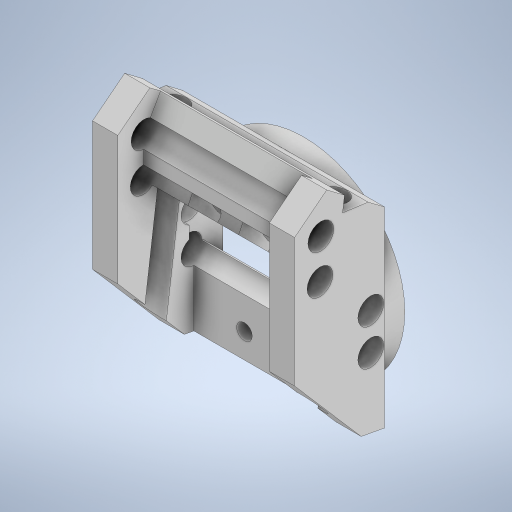
# Autodesk Inventor part: arm_head_top
Saved by Autodesk Inventor 2023.4 (Build 274418000, 418)
## iProperties
Created: 2024-03-10
Part Number: arm_head_top
Material: Generic
Document SubType Name: Modeling
Designer: aaron
Density: 1 g/cm^3
Appearance: Default
Author: aaron
Autodesk Inventor part; units mm, degrees
ref_plane "YZ Plane" through (0, 0, 0) normal (1, 0, 0) x (0, 1, 0)
ref_plane "XZ Plane" through (0, 0, 0) normal (0, 1, 0) x (-1, 0, 0)
sketch "Sketch1" plane through (0, 0, 0) normal (0, 0, 1) x (1, 0, 0)
  circle A0 centre (0, 0) radius 20
  dimension "d0" = 40
  constraints: 1 centre point, 1 coincident
  measures "d0" diameter of A0
extrude "Extrusion1" add sketch "Sketch1" along normal blind 4
sketch "Sketch2" plane through (0, 0, 0) normal (1, 0, 0) x (0, 1, 0)
  circle A0 centre (3.6, 6.738761) radius 2.55
  circle A1 centre (13.561537, 16.796235) radius 2.55
  circle A2 centre (21.281943, 16.626298) radius 2.55
  line L0 (20, 4) -> (-20, 4)
  line L1 (20, 4) -> (28.645843, 15.452424)
  line L2 (28.645843, 15.452424) -> (23.66832, 21.807503)
  circle A3 centre (-3.6, 6.738761) radius 2.55
  line L3 (23.66832, 21.807503) -> (-1.788198, 21.807503)
  line L4 (-1.788198, 21.807503) -> (-17.016826, 8.639245)
  line L5 (-17.016826, 8.639245) -> (-17.886444, 4)
  line L6 (28.119895, 11.661622) -> (-16.306899, 17.559025)
  line L7 (25.778694, 6.827665) -> (-17.950211, 12.632428)
  line L8 (22.466619, 7.267324) -> (23.137728, 12.322976)
  point P0 (0, 0)
  point P1 (0, 4)
  point P2 (25.996794, 11.943451)
  dimension "d3" = 5.1
  dimension "d4" = 5.1
  dimension "d5" = 5.1
  dimension "d7" = 5.1
  dimension "d8" = 3.6
  dimension "d9" = 3.6
  dimension "d14" = 5.1
  constraints: 16 end point, 4 centre point, 4 point on line, 1 horizontal, 1 midpoint, 1 parallel, 1 perpendicular
  measures "d3" diameter of A0
  measures "d4" diameter of A1
  measures "d5" diameter of A2
  measures "d7" diameter of A3
  measures "d8" horizontal distance of point (0, 4) A3.centre
  measures "d9" horizontal distance of point (0, 4) A0.centre
  measures "d14" distance between parallel lines of L7 L6
extrude "Extrusion2" add sketch "Sketch2" along normal mid plane 40 contours L0 L5 L4 L7 L1 | L7 L4 L6 L8 | L6 L4 L3 L2 L1
sketch "Sketch3" plane through (0, 0, 0) normal (1, 0, 0) x (0, 1, 0)
  circle A0 centre (21.281943, 16.626298) radius 2.55
  line L0 (30.616324, 11.312456) -> (21.281943, 16.626298)
  circle A1 centre (13.561537, 16.796235) radius 2.55
  line L1 (21.281943, 13.244246) -> (13.561537, 13.244246)
  circle A2 centre (3.6, 6.738761) radius 2.55
  line L2 (13.561537, 16.796235) -> (3.6, 6.738761)
  circle A3 centre (-3.6, 6.738761) radius 2.55
  line L3 (3.6, 6.738761) -> (-3.6, 6.738761)
  line L4 (-3.6, 6.738761) -> (-17.923849, 6.738761)
  line L5 (-17.923849, 6.738761) -> (-11.412077, 27.137294)
  line L6 (-11.412077, 27.137294) -> (40.472491, 29.35639)
  line L7 (40.472491, 29.35639) -> (30.616324, 11.312456)
  point P0 (0, 0)
  point P1 (-6.15, 6.738761)
  point P2 (-1.05, 6.738761)
  point P3 (1.05, 6.738761)
  point P4 (5.394461, 8.550503)
  point P5 (11.767077, 14.984493)
  point P6 (16.11092, 16.74012)
  point P7 (18.73256, 16.682413)
  point P8 (23.498015, 15.364741)
  constraints: 14 end point, 1 horizontal, 1 point on line, 3 other
sketch "Sketch3 outline for Extrusion3" plane through (0, 0, 0) normal (1, 0, 0) x (0, 1, 0)
  line L0 (30.616324, 11.312456) -> (40.472491, 29.35639)
  line L1 (23.498015, 15.364741) -> (30.616324, 11.312456)
  arc A0 (18.73256, 16.682413) -> (23.498015, 15.364741) centre (21.281943, 16.626298) cw
  line L2 (16.11092, 16.74012) -> (18.73256, 16.682413)
  arc A1 (11.767077, 14.984493) -> (16.11092, 16.74012) centre (13.561537, 16.796235) cw
  line L3 (5.394461, 8.550503) -> (11.767077, 14.984493)
  arc A2 (1.05, 6.738761) -> (5.394461, 8.550503) centre (3.6, 6.738761) cw
  line L4 (-1.05, 6.738761) -> (1.05, 6.738761)
  arc A3 (-6.15, 6.738761) -> (-1.05, 6.738761) centre (-3.6, 6.738761) cw
  line L5 (-17.923849, 6.738761) -> (-6.15, 6.738761)
  line L6 (-11.412077, 27.137294) -> (-17.923849, 6.738761)
  line L7 (40.472491, 29.35639) -> (-11.412077, 27.137294)
extrude "Extrusion3" cut sketch "Sketch3 outline for Extrusion3" along normal mid plane 30
sketch "Sketch4" plane through (-20, 23.137728, 12.322976) normal (0, 0.9913042, -0.13159) x (1, 0, 0)
  circle A0 centre (35.8, 2.441814) radius 2.55
  line L0 (20, 15.260511) -> (20, -13.845546)
  circle A1 centre (4.2, 2.441814) radius 2.55
  dimension "d15" = 5.1
  dimension "d18" = 15.8
  constraints: 2 centre point, 2 end point, 1 symmetric about line, 1 vertical, 1 other
  measures "d15" diameter of A0
  measures "d18" distance from line of A0.centre L0
extrude "Extrusion4" cut sketch "Sketch4" against normal through all
sketch "Sketch5" plane through (0, 0, 0) normal (1, 0, 0) x (0, 1, 0)
  line L0 (-4.609838, 7.650021) -> (6.320462, 7.650021)
  circle A0 centre (-3.6, 6.738761) radius 2.55
  line L1 (-4.609838, 7.650021) -> (-3.6, 6.738761)
  line L2 (-3.6, 6.738761) -> (-3.6, -1.829044)
  circle A1 centre (3.6, 6.738761) radius 2.55
  line L3 (6.320462, 7.650021) -> (3.6, 6.738761)
  line L4 (3.6, 6.738761) -> (3.6, -1.829044)
  line L5 (3.6, -1.829044) -> (-3.6, -1.829044)
  point P0 (0, 0)
  constraints: 12 end point, 2 vertical, 1 horizontal, 1 perpendicular
extrude "Extrusion5" cut sketch "Sketch5" along normal mid plane 32 contours L0 A0 L2 L1 | L0 A1 L4 L5 L2 A0 | L0 A1 L3 L4 | L0 L3 A1 picked at (-3.14274, 7.346268)
chamfer "Chamfer1" distance 3.9 angle 45 2 edges at (0, -3.6, 0) (0, 3.6, 0)
sketch "Sketch6" plane through (0, 0, 0) normal (0, 0, -1) x (-1, 0, 0)
  circle A0 centre (5, -12.5) radius 1.55
  circle A1 centre (-5, -12.5) radius 1.55
  circle A2 centre (-5, 12.5) radius 1.55
  circle A3 centre (5, 12.5) radius 1.55
  circle A4 centre (0, 0) radius 16
  point P0 (11.969428, -9.066958)
  constraints: 5 centre point
extrude "Extrusion6" cut sketch "Sketch6" against normal through all contours A0 | A1 | A2 | A3
ref_plane "Work Plane1" through (0, 0, 11) normal (0, 0, -1) x (-1, 0, 0)
sketch "Sketch7" plane through (0, 0, 11) normal (0, 0, -1) x (-1, 0, 0)
  circle A0 centre (-5, 12.5) radius 1.55 projected
  circle A1 centre (-5, 12.5) radius 3
  circle A2 centre (5, 12.5) radius 1.55 projected
  circle A3 centre (5, 12.5) radius 3
  point P0 (0, 0)
  dimension "d27" = 6
  dimension "d28" = 6
  constraints: 2 centre point, 2 coincident
  measures "d27" diameter of A1
  measures "d28" diameter of A3
extrude "Extrusion7" cut sketch "Sketch7" against normal blind 10 contours A0 | A1 | A2 | A3
sketch "Sketch8" plane through (0, 0, 0) normal (0, 0, -1) x (-1, 0, 0)
  circle A0 centre (-5, 12.5) radius 1.55 projected
  circle A1 centre (-5, 12.5) radius 3
  circle A2 centre (-5, 12.5) radius 1.55 projected
  circle A3 centre (5, 12.5) radius 1.55 projected
  circle A4 centre (5, -12.5) radius 1.55 projected
  circle A5 centre (-5, -12.5) radius 1.55 projected
  circle A6 centre (5, 12.5) radius 3
  circle A7 centre (5, -12.5) radius 3
  circle A8 centre (-5, -12.5) radius 3
  point P0 (0, 0)
  dimension "d31" = 6
  dimension "d32" = 6
  dimension "d33" = 6
  dimension "d34" = 6
  constraints: 4 centre point, 4 coincident
  measures "d31" diameter of A1
  measures "d32" diameter of A6
  measures "d33" diameter of A7
  measures "d34" diameter of A8
extrude "Extrusion8" add sketch "Sketch8" along normal blind 2.9
chamfer "Chamfer2" distance 1 angle 45 4 edges at (8, 12.5, -2.9) (-2, 12.5, -2.9) (-2, -12.5, -2.9) (8, -12.5, -2.9)
equation "\"d4\" = d3"
equation "\"d5\" = d3"
equation "\"d7\" = d3"
equation "\"d9\" = d8"
equation "\"d14\" = d3"
body "Solid1"
